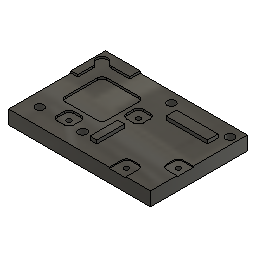
BracketProd_Fixture v2 (Autodesk Fusion 360 design; units mm, degrees)
Autodesk Fusion 360 part; units mm, degrees
sketch "Skizze1" plane through (0, 0, 0) normal (0, 1, 0) x (1, 0, 0)
  line L0 (0, 0) -> (102.5, 0)
  line L1 (102.5, 0) -> (102.5, -70)
  line L2 (102.5, -70) -> (0, -70)
  line L3 (0, -70) -> (0, 0)
  line L4 (0, 0) -> (5, 0)
  line L5 (5, 0) -> (5, -25)
  line L6 (5, -25) -> (0, -25)
  line L7 (0, -25) -> (0, 0)
  line L8 (0, 0) -> (25, 0)
  line L9 (25, 0) -> (25, -7.5)
  line L10 (25, -7.5) -> (0, -7.5)
  line L11 (0, -7.5) -> (0, 0)
  circle A0 centre (5, -7.5) radius 4
  circle A1 centre (27.5, -53.8) radius 1.65
  circle A2 centre (51.3, -27.5) radius 1.65
  line L12 (55.1, -25.926) -> (52.874, -23.7)
  line L13 (52.874, -23.7) -> (49.726, -23.7)
  line L14 (49.726, -23.7) -> (47.5, -25.926)
  line L15 (47.5, -25.926) -> (47.5, -29.074)
  line L16 (47.5, -29.074) -> (49.726, -31.3)
  line L17 (49.726, -31.3) -> (52.874, -31.3)
  line L18 (52.874, -31.3) -> (55.1, -29.074)
  line L19 (55.1, -29.074) -> (55.1, -25.926)
  line L20 (31.3, -52.226) -> (29.074, -50)
  line L21 (29.074, -50) -> (25.926, -50)
  line L22 (25.926, -50) -> (23.7, -52.226)
  line L23 (23.7, -52.226) -> (23.7, -55.374)
  line L24 (23.7, -55.374) -> (25.926, -57.6)
  line L25 (25.926, -57.6) -> (29.074, -57.6)
  line L26 (29.074, -57.6) -> (31.3, -55.374)
  line L27 (31.3, -55.374) -> (31.3, -52.226)
  line L28 (57.3, -21.5) -> (45.3, -21.5)
  line L29 (45.3, -21.5) -> (45.3, -33.5)
  line L30 (45.3, -33.5) -> (57.3, -33.5)
  line L31 (57.3, -33.5) -> (57.3, -21.5)
  line L32 (57.3, -21.5) -> (45.3, -33.5) construction
  line L33 (45.3, -21.5) -> (57.3, -33.5) construction
  line L34 (33.5, -47.8) -> (21.5, -47.8)
  line L35 (21.5, -47.8) -> (21.5, -59.8)
  line L36 (21.5, -59.8) -> (33.5, -59.8)
  line L37 (33.5, -59.8) -> (33.5, -47.8)
  line L38 (33.5, -47.8) -> (21.5, -59.8) construction
  line L39 (21.5, -47.8) -> (33.5, -59.8) construction
  circle A3 centre (55, -7.5) radius 3
  circle A4 centre (10, -57.5) radius 3
  line L40 (48.8, -40) -> (53.8, -40)
  line L41 (53.8, -40) -> (53.8, -60)
  line L42 (53.8, -60) -> (48.8, -60)
  line L43 (48.8, -60) -> (48.8, -40)
  line L44 (63.8, -12.5) -> (93.8, -12.5)
  line L45 (93.8, -12.5) -> (93.8, -20)
  line L46 (93.8, -20) -> (63.8, -20)
  line L47 (63.8, -20) -> (63.8, -12.5)
  line L48 (77.226, -60) -> (75, -62.226)
  circle A5 centre (78.8, -63.8) radius 1.65
  line L49 (75, -65.374) -> (77.226, -67.6)
  line L50 (80.374, -67.6) -> (82.6, -65.374)
  line L51 (72.8, -57.55) -> (72.8, -70.05)
  line L52 (75, -62.226) -> (75, -65.374)
  line L53 (84.8, -70.05) -> (84.8, -57.55)
  line L54 (84.8, -57.55) -> (72.8, -57.55)
  line L55 (72.8, -57.55) -> (84.8, -70.05) construction
  line L56 (82.6, -62.226) -> (80.374, -60)
  line L57 (77.226, -67.6) -> (80.374, -67.6)
  line L58 (80.374, -60) -> (77.226, -60)
  line L59 (82.6, -65.374) -> (82.6, -62.226)
  line L60 (72.8, -70.05) -> (84.8, -70.05)
  line L61 (84.8, -57.55) -> (72.8, -70.05) construction
  line L62 (96.026, -41.2) -> (93.8, -43.426)
  circle A6 centre (97.6, -45) radius 1.65
  line L63 (93.8, -46.574) -> (96.026, -48.8)
  line L64 (99.174, -48.8) -> (101.4, -46.574)
  line L65 (91.6, -39) -> (91.6, -51)
  line L66 (93.8, -43.426) -> (93.8, -46.574)
  line L67 (103.6, -51) -> (103.6, -39)
  line L68 (103.6, -39) -> (91.6, -39)
  line L69 (91.6, -39) -> (103.6, -51) construction
  line L70 (101.4, -43.426) -> (99.174, -41.2)
  line L71 (96.026, -48.8) -> (99.174, -48.8)
  line L72 (99.174, -41.2) -> (96.026, -41.2)
  line L73 (101.4, -46.574) -> (101.4, -43.426)
  line L74 (91.6, -51) -> (103.6, -51)
  line L75 (103.6, -39) -> (91.6, -51) construction
  line L76 (42.5, -15) -> (12.5, -15)
  line L77 (12.5, -15) -> (12.5, -45)
  line L78 (12.5, -45) -> (42.5, -45)
  line L79 (42.5, -45) -> (42.5, -15)
  line L80 (42.5, -15) -> (12.5, -45) construction
  line L81 (12.5, -15) -> (42.5, -45) construction
  circle A7 centre (41, -57.5) radius 3
  circle A8 centre (97.5, -7.5) radius 3
  point P0 (51.3, -27.5)
  point P1 (27.5, -53.8)
  point P2 (51.3, -27.5)
  point P3 (27.5, -53.8)
  point P4 (78.8, -63.8)
  point P5 (78.8, -63.8)
  point P6 (97.6, -45)
  point P7 (97.6, -45)
  point P8 (27.5, -30)
  dimension "d1" = 102.5
  dimension "d2" = 70
  dimension "d3" = 5
  dimension "d4" = 25
  dimension "d5" = 25
  dimension "d6" = 7.5
  dimension "d7" = 8
  dimension "d8" = 3.3
  dimension "d9" = 46.3
  dimension "d11" = 3.3
  dimension "d13" = 46.3
  dimension "d14" = 20
  dimension "d15" = 22.5
  dimension "d16" = 3.8
  dimension "d17" = 3.8
  dimension "d18" = 12
  dimension "d19" = 12
  dimension "d20" = 12
  dimension "d21" = 12
  dimension "d34" = 6
  dimension "d35" = 6
  dimension "d36" = 7.5
  dimension "d37" = 55
  dimension "d38" = 50
  dimension "d39" = 10
  dimension "d40" = 5
  dimension "d41" = 20
  dimension "d42" = 2.5
  dimension "d43" = 60
  dimension "d44" = 30
  dimension "d45" = 7.5
  dimension "d47" = 10
  dimension "d48" = 3.3
  dimension "d49" = 3.8
  dimension "d50" = 12
  dimension "d51" = 12.5
  dimension "d52" = 43.8
  dimension "d53" = 15
  dimension "d54" = 3.3
  dimension "d55" = 3.8
  dimension "d56" = 12
  dimension "d57" = 12
  dimension "d58" = 43.8
  dimension "d59" = 15
  dimension "d84" = 20
  dimension "d85" = 30
  dimension "d86" = 30
  dimension "d87" = 22.5
  dimension "d88" = 22.5
  dimension "d131" = 6
  dimension "d132" = 50
  dimension "d133" = 31
  dimension "d134" = 6
  dimension "d135" = 7.5
  dimension "d136" = 5
  constraint horizontal L0
  constraint vertical L1
  constraint horizontal L2
  constraint vertical L3
  constraint coincident L0.start L3.end
  constraint horizontal L4
  constraint vertical L5
  constraint horizontal L6
  constraint vertical L7
  constraint horizontal L8
  constraint vertical L9
  constraint horizontal L10
  constraint vertical L11
  constraint coincident L10 A0.centre
  constraint coincident L5 A0.centre
  constraint coincident P2 P0
  constraint coincident P3 P1
  constraint horizontal L28
  constraint perpendicular L28 L29
  constraint parallel L28 L30
  constraint parallel L29 L31
  constraint coincident L32 P2
  constraint coincident L33 P2
  constraint parallel L2 L25
  constraint parallel L17 L25
  constraint horizontal L34
  constraint perpendicular L34 L35
  constraint parallel L34 L36
  constraint parallel L35 L37
  constraint coincident L38 P3
  constraint coincident L39 P3
  constraint horizontal L40
  constraint vertical L41
  constraint horizontal L42
  constraint vertical L43
  constraint horizontal L44
  constraint vertical L45
  constraint horizontal L46
  constraint vertical L47
  constraint coincident P5 P4
  constraint horizontal L54
  constraint perpendicular L51 L54
  constraint parallel L54 L60
  constraint parallel L51 L53
  constraint coincident P5 L61
  constraint coincident P5 L55
  constraint parallel L2 L57
  constraint coincident P7 P6
  constraint horizontal L68
  constraint perpendicular L65 L68
  constraint parallel L68 L74
  constraint parallel L65 L67
  constraint coincident P7 L75
  constraint coincident P7 L69
  constraint parallel L57 L71
  constraint horizontal L76
  constraint perpendicular L76 L77
  constraint parallel L76 L78
  constraint parallel L77 L79
  constraint coincident L80 P8
  constraint coincident L81 P8
  measures "d1" distance of L0.start L0.end
  measures "d2" distance of L0.start L2.end
  measures "d3" distance of L0.start L4.end
  measures "d4" distance of L0.start L6.end
  measures "d5" distance of L0.start L8.end
  measures "d6" distance of L0.start L10.end
  measures "d7" diameter of A0
  measures "d8" diameter of A1
  measures "d9" distance of L10 P3
  measures "d11" diameter of A2
  measures "d13" distance of L5 P2
  measures "d14" vertical distance of L9.end P2
  measures "d15" horizontal distance of L5.end P3
  measures "d16" distance of P2 L19
  measures "d17" distance of P3 L27
  measures "d18" distance of L29.end L30.end
  measures "d19" distance of L28.end L29.end
  measures "d20" distance of L35.end L36.end
  measures "d21" distance of L34.end L35.end
  measures "d34" diameter of A3
  measures "d35" diameter of A4
  measures "d36" distance of L0 A3.centre
  measures "d37" distance of L3 A3.centre
  measures "d38" vertical distance of A3.centre A4.centre
  measures "d39" distance of L3 A4.centre
  measures "d40" distance of L40.start L40.end
  measures "d41" distance of L40.start L42.end
  measures "d42" horizontal distance of P2 L40.end
  measures "d43" distance of L0 L42
  measures "d44" distance of L44.start L44.end
  measures "d45" distance of L44.start L46.end
  measures "d47" horizontal distance of L40.end L46.end
  measures "d48" diameter of A5
  measures "d49" distance of P5 L59
  measures "d50" distance of L51.end L53.start
  measures "d51" distance of L51.end L51.start
  measures "d52" distance of L46 P5
  measures "d53" horizontal distance of L45.end P5
  measures "d54" diameter of A6
  measures "d55" distance of P7 L73
  measures "d56" distance of L65.end L67.start
  measures "d57" distance of L65.end L65.start
  measures "d58" distance of L41 P7
  measures "d59" vertical distance of L41.end P7
  measures "d84" vertical distance of L40.end L46.end
  measures "d85" distance of L77.end L78.end
  measures "d86" distance of L76.end L77.end
  measures "d87" horizontal distance of A0.centre P8
  measures "d88" distance of L10 P8
  measures "d131" diameter of A7
  measures "d132" vertical distance of A3.centre A7.centre
  measures "d133" distance of A4.centre A7.centre
  measures "d134" diameter of A8
  measures "d135" distance of L0 A8.centre
  measures "d136" distance of L1 A8.centre
extrude "Extrusion1" add sketch "Skizze1" against normal blind 10 contours L0 L3 L4 L5 L7 L8 L10 L11 A0 | L0 L5 L8 L9 L10 A0 | L3 L5 L6 L7 L10 A0 | L0 L1 L2 L3 L5 L6 L9 L10 A0 L51 L53 L54 L65 L68 L74 | L5 L10 A0 | L5 L10 A0 | L5 L10 A0 | L5 L10 A0 | L1 L65 L68 L74 | L2 L51 L53 L54 | L12 L13 L14 L15 L16 L17 L18 L19 | L20 L21 L22 L23 L24 L25 L26 L27 | L28 L29 L30 L31 | L34 L35 L36 L37 | L40 L41 L42 L43 | L44 L45 L46 L47 | L48 L49 L50 L52 L56 L57 L58 L59 | L62 L63 L64 L66 L70 L71 L72 L73 | L76 L77 L78 L79 makes body 1
extrude "Extrusion2" add sketch "Skizze1" along normal blind 1.5 contours L0 L3 L4 L5 L7 L8 L10 L11 A0 | L0 L5 L8 L9 L10 A0 | L3 L5 L6 L7 L10 A0 bodies 1
extrude "Extrusion3" cut sketch "Skizze1" against normal blind 1.5 contours A1 | A2 | L12 L13 L14 L15 L16 L17 L18 L19 | L20 L21 L22 L23 L24 L25 L26 L27 | L28 L29 L30 L31 | L34 L35 L36 L37 | L76 L77 L78 L79 bodies 1
extrude "Extrusion5" add sketch "Skizze1" along normal blind 2.5 contours L40 L41 L42 L43 | L44 L45 L46 L47 bodies 1
extrude "Extrusion6" cut sketch "Skizze1" against normal blind 0.8 contours L1 L67 L68 L74 | L1 L65 L68 L74 | L2 L51 L53 L54 | L2 L51 L53 L60 | L48 L49 L50 L52 L56 L57 L58 L59 | L62 L63 L64 L66 L70 L71 L72 L73 bodies 1
fillet "Abrundung1" radius 3.5 10 edges at (21.5, -0.75, 59.8) (45.3, -0.75, 33.5) (57.3, -0.75, 33.5) (33.5, -0.75, 59.8) (57.3, -0.75, 21.5) (33.5, -0.75, 47.8) (45.3, -0.75, 21.5) (21.5, -0.75, 47.8) (9, 0.75, 7.5) (5, 0.75, 11.5) on bodies 1
fillet "Abrundung1" radius 3.5 7 edges at (42.5, -0.75, 15) (42.5, -0.75, 45) (12.5, -0.75, 45) (12.5, -0.75, 15) (72.8, -0.4, 57.55) (91.6, -0.4, 39) (84.8, -0.4, 57.55) on bodies 1
fillet "Abrundung1" radius 3.5 1 edges at (91.6, -0.4, 51) on bodies 1
copy_body "Körper->Berechn1" bodies 1 removing the originals makes body 2 in component "Fixture"
component "Fixture" placed x (1, 0, 0) y (0, 1, 0) z (0, 0, 1) at (0, 0, 0)
equation "d9 = 3.8 mm + 42.5 mm"
equation "d13 = d9"
equation "d52 = 40 mm + 3.8 mm"
equation "d58 = d52"
equation "d62 = -2.8 mm + 2 mm"
equation "d132 = d38"
